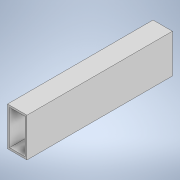
# Autodesk Inventor part: C_358_40_2
Saved by Autodesk Inventor 2020 (Build 240168000, 168)
## iProperties
Created: 2022-03-28
Part Number: C_358_40_2
Material: Genérico
Document SubType Name: Modeling
Designer: aarco
Density: 1 g/cm^3
Appearance: Valor por defecto
Author: aarco
Autodesk Inventor part; units mm, degrees
ref_plane "YZ Plane" through (0, 0, 0) normal (1, 0, 0) x (0, 1, 0)
ref_plane "XZ Plane" through (0, 0, 0) normal (0, 1, 0) x (-1, 0, 0)
ref_plane "XY Plane" through (0, 0, 0) normal (0, 0, 1) x (1, 0, 0)
sketch "Boceto1" plane through (0, 0, 0) normal (0, 0, 1) x (1, 0, 0)
  line L0 (-10, 20) -> (10, 20)
  line L1 (10, 20) -> (10, -20)
  line L2 (10, -20) -> (-10, -20)
  line L3 (-10, -20) -> (-10, 20)
  line L4 (-10, 20) -> (10, -20) construction
  line L5 (6.3055, 0) -> (10, 0) construction
  line L6 (0, -12.611) -> (0, -20) construction
  line L7 (-8, 18) -> (8, 18)
  line L8 (8, 18) -> (8, -18)
  line L9 (8, -18) -> (-8, -18)
  line L10 (-8, -18) -> (-8, 18)
  line L11 (-8, 0) -> (-10, 0)
  line L12 (0, 18) -> (0, 20)
  point P0 (0, 0)
  point P1 (0, 0)
  dimension "d0" = 40
  dimension "d4" = 20
  dimension "d5" = 2
  dimension "d6" = 2
  constraints: 26 end point, 7 midpoint, 5 perpendicular, 4 parallel, 2 horizontal, 1 coincident
  measures "d0" distance of L2.end L0.start
  measures "d4" distance of L0.start L0.end
  measures "d5" distance between parallel lines of L0 L7
  measures "d6" distance between parallel lines of L3 L10
extrude "Extrusión1" add sketch "Boceto1" along normal blind 150 contours L0 L12 L7 L10 L11 L3 | L0 L1 L2 L3 L11 L10 L9 L8 L7 L12
